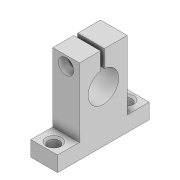
# Autodesk Inventor part: SK16
Saved by Autodesk Inventor 2020 (Build 240168000, 168)
## iProperties
Created: 2021-10-09
Part Number: SK16
Material: Generic
Document SubType Name: Modeling
Designer: Henry Cawley
Density: 1 g/cm^3
Appearance: Default
Author: Henry Cawley
Autodesk Inventor part; units mm, degrees
ref_plane "YZ Plane" through (0, 0, 0) normal (1, 0, 0) x (0, 1, 0)
ref_plane "XZ Plane" through (0, 0, 0) normal (0, 1, 0) x (-1, 0, 0)
ref_plane "XY Plane" through (0, 0, 0) normal (0, 0, 1) x (1, 0, 0)
sketch "Sketch1" plane through (0, 0, 0) normal (1, 0, 0) x (0, 1, 0)
  line L0 (0, 0) -> (0, -48)
  line L1 (0, -48) -> (8, -48)
  line L2 (8, -48) -> (8, -36.5)
  line L3 (8, -36.5) -> (44, -36.5)
  line L4 (44, -36.5) -> (44, -11.5)
  line L5 (44, -11.5) -> (8, -11.5)
  line L6 (8, -11.5) -> (8, 0)
  line L7 (8, 0) -> (0, 0)
  circle A0 centre (27, -24) radius 8
  dimension "d0" = 8
  dimension "d1" = 48
  dimension "d2" = 11.5
  dimension "d3" = 11.5
  dimension "d4" = 44
  dimension "d5" = 16
  dimension "d6" = 17
  dimension "d7" = 12.5
  constraints: 16 end point, 6 perpendicular, 2 point on line, 1 centre point, 1 vertical
  measures "d0" distance of L6.end L0.start
  measures "d1" distance of L0.start L0.end
  measures "d2" distance of L5.end L6.end
  measures "d3" distance of L1.end L2.end
  measures "d4" distance between parallel lines of L0 L4
  measures "d5" diameter of A0
  measures "d6" distance from line of L4 A0.centre
  measures "d7" distance from line of L5 A0.centre
extrude "Extrusion1" add sketch "Sketch1" along normal blind 14
sketch "Sketch2" plane through (14, 0, 0) normal (1, 0, 0) x (0, 0, -1)
  line L0 (36.5, 44) -> (11.5, 44) projected
  line L1 (22.5, 44) -> (24.5, 44)
  line L2 (24.5, 44) -> (24.5, 26.6332)
  line L3 (24.5, 26.6332) -> (22.5, 26.6332)
  line L4 (22.5, 26.6332) -> (22.5, 44)
  line L5 (11.5, 44) -> (11.5, 8) projected
  point P0 (0, 0)
  dimension "d10" = 2
  dimension "d12" = 11
  constraints: 8 end point, 2 parallel, 1 horizontal, 1 perpendicular, 1 point on line
  measures "d10" distance of L2.end L3.end
  measures "d12" distance between parallel lines of L5 L4
extrude "Extrusion2" cut sketch "Sketch2" against normal blind 33.25
sketch "Sketch3" plane through (0, 8, -11.5) normal (0, 0, 1) x (1, 0, 0)
  circle A0 centre (7, 31) radius 2
  line L0 (0, 36) -> (14, 36) projected
  line L1 (0, 36) -> (0, 0) projected
  point P0 (0, -8)
  dimension "d15" = 5
  dimension "d16" = 7
  dimension "d17" = 4
  constraints: 1 centre point
  measures "d15" distance from line of L0 A0.centre
  measures "d16" distance from line of L1 A0.centre
  measures "d17" diameter of A0
extrude "Extrusion3" cut sketch "Sketch3" against normal blind 33.25
sketch "Sketch4" plane through (0, 8, 0) normal (0, 1, 0) x (1, 0, 0)
  circle A0 centre (7, 5) radius 3
  circle A1 centre (7, 43) radius 3
  line L0 (14, 11.5) -> (14, 0) projected
  line L1 (14, 48) -> (14, 36.5) projected
  line L2 (0, 0) -> (14, 0) projected
  line L3 (0, 48) -> (14, 48) projected
  dimension "d20" = 6
  dimension "d21" = 7
  dimension "d22" = 7
  dimension "d23" = 5
  dimension "d24" = 5
  constraints: 2 centre point, 1 equal radius
  measures "d20" diameter of A0
  measures "d21" distance from line of L0 A0.centre
  measures "d22" distance from line of L1 A1.centre
  measures "d23" distance from line of L2 A0.centre
  measures "d24" distance from line of L3 A1.centre
extrude "Extrusion4" cut sketch "Sketch4" against normal blind 33.25
chamfer "Chamfer1" distance 1 angle 45 2 edges at (4, 8, -5) (4, 8, -43)
sketch "Sketch5" plane through (0, 8, -11.5) normal (0, 0, 1) x (1, 0, 0)
  circle A0 centre (7, 31) radius 2 projected
  circle A1 centre (7, 31) radius 4
  point P0 (0, -8)
  dimension "d30" = 8
  constraints: 1 centre point, 1 coincident
  measures "d30" diameter of A1
extrude "Extrusion5" cut sketch "Sketch5" against normal blind 5
thread "Thread1" size "M4x0.7" class "6H" standard "ANSI Metric M Profile" length 10
body "Solid1"
